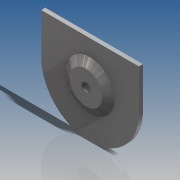
# Autodesk Inventor part: 56555-ElectricAlloy
Saved by Autodesk Inventor 2016 SP2 (Build 200236200, 236)
## iProperties
Created: 2015-08-19
Part Number: 56555-ElectricAlloy
Material: Steel
Document SubType Name: Modeling
Designer: D. Kohfeld
Density: 7.85 g/cm^3
Appearance: ElectricAlloy
Mass: 0.273659 g
Surface Area: 1.63558 cm^2
Volume: 0.034861 cm^3
Author: D. Kohfeld
Autodesk Inventor part; units mm, degrees
ref_plane "YZ Plane" through (0, 0, 0) normal (1, 0, 0) x (0, 1, 0)
ref_plane "XZ Plane" through (0, 0, 0) normal (0, 1, 0) x (-1, 0, 0)
ref_plane "XY Plane" through (0, 0, 0) normal (0, 0, 1) x (1, 0, 0)
sketch "Sketch2" plane through (0, 0, 0) normal (0, 0, 1) x (1, 0, 0)
  line L0 (-4.8, 4) -> (-4.8, 0)
  arc A0 (-4.8, 0) -> (4.8, 0) centre (0, 0) ccw
  line L1 (4.8, 0) -> (4.8, 4)
  line L2 (4.8, 4) -> (-4.8, 4)
  dimension "d0" = 9.6
  dimension "d1" = 8.8
  constraints: 6 end point, 2 point on circle, 2 tangent, 2 vertical, 1 centre point, 1 coincident, 1 horizontal
  measures "d0" distance of L1.end L0.start
extrude "Extrusion1" add sketch "Sketch2" against normal blind 0.4
sketch "Sketch3" plane through (0, 0, 0) normal (1, 0, 0) x (0, 1, 0)
  line L0 (-0.4, 0.4) -> (-1.6, 0.4)
  line L1 (-1.6, 0.4) -> (-2.4, 0)
  line L2 (-2.4, 0) -> (0, 0)
  line L3 (0, 0) -> (0, 0.2)
  ellipse E0 centre (0, 0.4) end of major axis (-0.4, 0.4) minor radius 0.2 (-0.4, 0.4) -> (0, 0.2) ccw
  dimension "d4" = 0.8
  dimension "d5" = 0.2
  dimension "d6" = 0.4
  dimension "d7" = 3.2
  dimension "d8" = 4.8
  constraints: 8 end point, 2 horizontal, 1 horizontal alignment, 1 vertical, 1 vertical alignment, 4 other
  measures "d4" diameter of L0.start L3
  measures "d5" distance from line of L3.end L0
  measures "d6" distance between parallel lines of L2 L0
  measures "d7" diameter of L0.end L3
  measures "d8" diameter of L1.end L3
revolve "Revolution1" add sketch "Sketch3" angle 360 about axis through (0, 0, 0) along (0, 0, 1)
fillet "Fillet1" radius 0.1 3 edges at (0, 1.6, 0.4) (0, 2.4, 0) (0, 0.4, 0.4)
body "Solid1"
